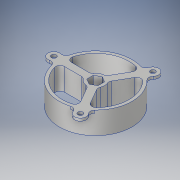
# Autodesk Inventor part: Flywheel Half
Saved by Autodesk Inventor 2019.4 (Build 234330000, 330)
## iProperties
Created: 2020-01-16
Part Number: Flywheel Half
Material: Aluminum 6061
Document SubType Name: Modeling
Designer: admin
Density: 2.7 g/cm^3
Appearance: Aluminum - Flat
Mass: 120.018 g
Surface Area: 219.742 cm^2
Volume: 44.4513 cm^3
Author: admin
Autodesk Inventor part; units mm, degrees
ref_plane "YZ Plane" through (0, 0, 0) normal (1, 0, 0) x (0, 1, 0)
ref_plane "XZ Plane" through (0, 0, 0) normal (0, 1, 0) x (-1, 0, 0)
ref_plane "XY Plane" through (0, 0, 0) normal (0, 0, 1) x (1, 0, 0)
sketch "Sketch1" plane through (0, 0, 0) normal (1, 0, 0) x (0, 1, 0)
  line L0 (12.5, 40.88) -> (7.5, 40.88)
  line L1 (-12.5, 40.88) -> (-12.5, 40.88) construction
  line L2 (-12.5, 0) -> (12.5, 0)
  line L3 (12.5, 0) -> (12.5, 40.88)
  line L4 (7.5, 40.88) -> (-12.5, 40.88)
  line L5 (7.5, 40.88) -> (-12.5, 40.88) construction
  line L6 (-12.5, 40.88) -> (-12.5, 0)
  point P0 (0, 0)
  point P1 (0, 0)
  dimension "d0" = 40.88
  dimension "d1" = 25
  dimension "d2" = 0
  dimension "d3" = 20
  constraints: 14 end point, 4 parallel, 4 perpendicular, 2 horizontal, 1 coincident, 1 midpoint
  measures "d0" distance of L2.end L0.start
  measures "d1" distance of L0.start L1.start
  measures "d2" vertical distance of L0.end L1.end
  measures "d3" distance of L0.end L1.end
revolve "Revolution1" add sketch "Sketch1" angle 360 about axis through (0, -12.5, 0) along (0, 1, 0)
sketch "Sketch2" plane through (0, -12.5, 0) normal (0, -1, 0) x (1, 0, 0)
  line L0 (-6.35, 3.6662) -> (0, 7.3323)
  line L1 (0, 7.3323) -> (6.35, 3.6662)
  line L2 (6.35, 3.6662) -> (6.35, -3.6662)
  line L3 (6.35, -3.6662) -> (0, -7.3323)
  line L4 (0, -7.3323) -> (-6.35, -3.6662)
  line L5 (-6.35, -3.6662) -> (-6.35, 3.6662)
  circle A0 centre (23, 0) radius 14
  line L6 (23, 0) -> (0, 0) construction
  circle A1 centre (23.3345, -23.3345) radius 6
  line L7 (0, 0) -> (23.3345, -23.3345) construction
  circle A2 centre (0, 23) radius 14
  circle A3 centre (23.3345, 23.3345) radius 6
  circle A4 centre (-23, 0) radius 14
  circle A5 centre (-23.3345, 23.3345) radius 6
  circle A6 centre (0, -23) radius 14
  circle A7 centre (-23.3345, -23.3345) radius 6
  circle A8 centre (0, 0) radius 37.5
  circle A9 centre (0, 0) radius 10
  line L8 (-4, 9.1652) -> (-4, 37.2861) construction
  line L9 (4, 9.1652) -> (4, 37.2861) construction
  point P0 (0, 0)
  dimension "d8" = 12.7
  dimension "d9" = 28
  dimension "d10" = 23
  dimension "d11" = 12
  dimension "d12" = 45
  dimension "d13" = 33
  dimension "d16" = 360
  dimension "d20" = 75
  dimension "d21" = 20
  dimension "d22" = 8
  constraints: 20 end point, 10 centre point, 4 point on circle, 3 coincident, 2 parallel, 2 vertical, 1 horizontal, 30 other
  measures "d8" distance between parallel lines of L2 L5
  measures "d9" diameter of A0
  measures "d10" distance of L6.start L6.end
  measures "d11" diameter of A1
  measures "d12" angle of L6 L7
  measures "d13" distance of L6.end L7.end
  measures "d20" diameter of A8
  measures "d21" diameter of A9
  measures "d22" distance between parallel lines of L8 L9
extrude "Extrusion1" cut sketch "Sketch2" against normal through all contours L0 L1 L2 L3 L4 L5 | A0 A9 | A9 A2 | A6 A9 | A9 A4 | A1 A8 | A1 A8 A7 A5 A3 | A8 A7 | A3 A8 | A8 A5 picked at (27.8646, 1.1161) picked at (-0.7795, 27.8977) picked at (-0.7795, -27.8977) picked at (-27.8426, -1.4978) picked at (24.2116, -23.8676) picked at (-23.9477, -24.1155) picked at (24.2116, 23.8676) picked at (-23.9477, 24.1155)
sketch "Sketch3" plane through (0, -12.5, 0) normal (0, -1, 0) x (1, 0, 0)
  line L0 (-9.1652, 4) -> (-37.2861, 4)
  circle A0 centre (0, 0) radius 10 projected
  circle A1 centre (0, 0) radius 37.5 projected
  line L1 (-9.1652, -4) -> (-37.2861, -4)
  circle A2 centre (0, 0) radius 37.5 projected
  point P0 (0, 0)
  dimension "d23" = 8
  constraints: 4 end point, 3 point on circle, 2 horizontal, 1 parallel, 2 other
  measures "d23" distance between parallel lines of L1 L0
extrude "Extrusion2" add sketch "Sketch3" against normal up to surface (25 mm away) contours A0 L1 A1 L0 picked at (-28.2541, -1.7785)
pattern_circular "Circular Pattern1" count 3 over 360 about axis through (0, -12.5, 0) along (0, 1, 0) of "Extrusion2"
fillet "Fillet1" radius 5 12 edges at (-9.1652, 0, -4) (1.1185, 0, -9.9373) (-9.1652, 0, 4) (1.1185, 0, 9.9373) (8.0467, 0, 5.9373) (8.0467, 0, -5.9373) (15.1789, 0, 34.2907) (22.1071, 0, 30.2907) (-37.2861, 0, -4) (-37.2861, 0, 4) (15.1789, 0, -34.2907) (22.1071, 0, -30.2907)
sketch "Sketch4" plane through (0, 12.5, 0) normal (0, 1, 0) x (1, 0, 0)
  circle A0 centre (-47.18, 0) radius 2.75
  circle A1 centre (-47.18, 0) radius 6.5
  circle A2 centre (0, 0) radius 40.88 projected
  line L0 (-47.18, 0) -> (0, 0) construction
  point P0 (0, 0)
  dimension "d32" = 5.5
  dimension "d33" = 13
  dimension "d34" = 47.18
  constraints: 2 centre point, 2 end point, 1 coincident, 1 horizontal
  measures "d32" diameter of A0
  measures "d33" diameter of A1
  measures "d34" distance of L0.start L0.end
extrude "Extrusion3" add sketch "Sketch4" against normal blind 3 contours A1 A2 | A2 A1 picked at (-40.8113, 0) picked at (-52.3399, -0.7397)
fillet "Fillet2" radius 5 2 edges at (-40.8529, 11, 1.4891) (-40.8529, 11, -1.4891)
pattern_circular "Circular Pattern2" count 3 over 360 about axis through (0, 10, 0) along (0, 1, 0) of "Extrusion3", "Fillet2"
body "Solid1"
